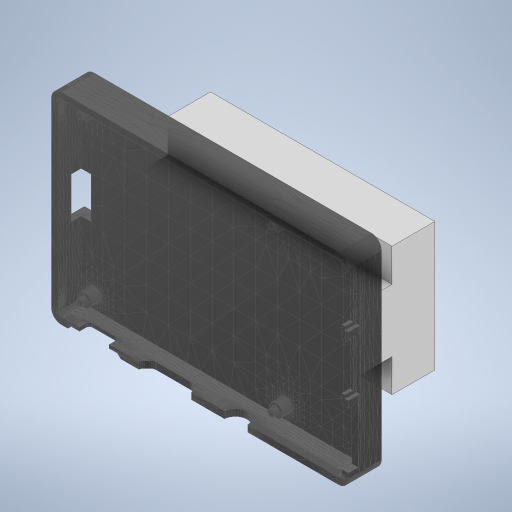
# Autodesk Inventor part: Inferior
Saved by Autodesk Inventor 2023 (Build 270158000, 158)
## iProperties
Created: 2022-06-21
Part Number: Inferior
Material: Generic
Document SubType Name: Modeling
Designer: nikol
Density: 1 g/cm^3
Appearance: Default
Author: nikol
Autodesk Inventor part; units mm, degrees
ref_plane "YZ Plane" through (0, 0, 0) normal (1, 0, 0) x (0, 1, 0)
ref_plane "XZ Plane" through (0, 0, 0) normal (0, 1, 0) x (-1, 0, 0)
ref_plane "XY Plane" through (0, 0, 0) normal (0, 0, 1) x (1, 0, 0)
sketch "Sketch1" plane through (-41, -6, 0) normal (0, 0, -1) x (-1, 0, 0)
  line L0 (-10.2196, -17.8058) -> (-78.2196, -17.8058)
  line L1 (-78.2196, -17.8058) -> (-78.2196, 29.1942)
  line L2 (-78.2196, 29.1942) -> (-10.2196, 29.1942)
  line L3 (-10.2196, 29.1942) -> (-10.2196, -17.8058)
  point P0 (-41, 6)
  dimension "d0" = 68
  dimension "d1" = 47
  constraints: 8 end point, 2 parallel, 1 horizontal, 1 perpendicular
  measures "d0" distance of L1.end L2.end
  measures "d1" distance of L0.end L1.end
extrude "Extrusion4" add sketch "Sketch1" along normal blind 30
sketch "Sketch5" plane through (-30.7804, -23.8058, 0) normal (-1, 0, 0) x (0, 0, 1)
  line L0 (0, 47) -> (0, 0) projected
  line L1 (0, 0) -> (0, 14)
  line L2 (0, 47) -> (0, 33)
  line L3 (0, 14) -> (-11, 14)
  line L4 (-11, 14) -> (-11, 4)
  line L5 (0, 33) -> (-11, 33)
  line L6 (-11, 33) -> (-11, 43)
  line L7 (-11, 4) -> (-24, 4)
  line L8 (-11, 43) -> (-24, 43)
  line L9 (-24, 43) -> (-24, 4)
  line L10 (0, 14) -> (0, 33)
  line L11 (0, 14) -> (0, 0)
  line L12 (0, 0) -> (-30, 0) projected
  line L13 (-30, 47) -> (-30, 0) projected
  line L14 (-30, 0) -> (-30, 47)
  line L15 (-30, 47) -> (0, 47)
  line L16 (0, 47) -> (0, 33)
  line L17 (0, 33) -> (0, 47)
  line L18 (-30, 0) -> (0, 0)
  line L19 (0, 0) -> (0, 14)
  line L20 (0, 0) -> (0, 47)
  point P0 (0, 23.8058)
  dimension "d32" = 14
  dimension "d33" = 14
  dimension "d34" = 11
  dimension "d35" = 10
  dimension "d36" = 11
  dimension "d37" = 10
  dimension "d38" = 13
  dimension "d39" = 13
  constraints: 36 end point, 7 collinear, 4 horizontal, 3 perpendicular, 2 point on line, 1 vertical
  measures "d32" distance of L0.end L1.end
  measures "d33" distance of L0.start L2.end
  measures "d34" distance of L1.end L3.end
  measures "d35" distance of L3.end L4.end
  measures "d36" distance of L2.end L5.end
  measures "d37" distance of L5.end L6.end
  measures "d38" distance of L4.end L7.end
  measures "d39" distance of L6.end L8.end
extrude "Extrusion5" cut sketch "Sketch5" against normal blind 68 contours L0 L5 L6 L8 L9 L7 L4 L3 L12 L13 L15
body "Solid2"
